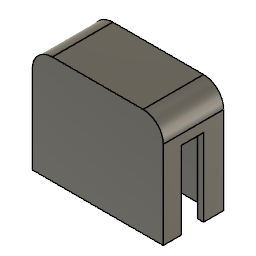
cover_motor_bottom (Autodesk Fusion 360 design; units mm, degrees)
Autodesk Fusion 360 part; units mm, degrees
sketch "Sketch1" plane through (0, 0, 0) normal (0, 1, 0) x (1, 0, 0)
  line L0 (25.6354, -40) -> (70.6354, -40)
  line L1 (80.6354, -30) -> (80.6354, 13.5)
  line L2 (80.6354, 13.5) -> (15.6354, 13.5)
  line L3 (15.6354, 13.5) -> (15.6354, -30)
  arc A0 (15.6354, -30) -> (25.6354, -40) centre (25.6354, -30) ccw
  arc A1 (70.6354, -40) -> (80.6354, -30) centre (70.6354, -30) ccw
  dimension "d1" = 65
  dimension "d2" = 53.5
  dimension "d3" = 10
  dimension "d4" = 10
  constraint horizontal L0
  constraint vertical L1
  constraint horizontal L2
  constraint vertical L3
  constraint tangent L0 A0
  constraint tangent L3 A0
  constraint tangent L0 A1
  constraint tangent L1 A1
  measures "d1" distance of L1 L3
  measures "d2" distance of L0 L2
  measures "d3" radius of A0
  measures "d4" radius of A1
extrude "Extrude2" add sketch "Sketch1" along normal blind 30
shell "Shell2" thickness 3 removed faces 1 at (58.9688, 20, -13.5)
sketch "Sketch3" plane through (80.6354, 0, 0) normal (1, 0, 0) x (0, 1, 0)
  line L0 (0, 30) -> (0, -13.5)
  line L1 (0, -13.5) -> (30, -13.5)
  line L2 (30, -13.5) -> (30, 30)
  line L3 (30, 30) -> (0, 30)
  line L4 (9, 25.0348) -> (20, 25.0348)
  line L5 (20, 25.0348) -> (20, -16.6958)
  line L6 (20, -16.6958) -> (9, -16.6958)
  line L7 (9, -16.6958) -> (9, 25.0348)
  dimension "d18" = 11
  constraint horizontal L4
  constraint vertical L5
  constraint horizontal L6
  constraint vertical L7
  measures "d18" distance of L5 L7
extrude "Extrude4" cut sketch "Sketch3" against normal blind 10 contours L1 L4 L5 L7 | L1 L5 L6 L7
